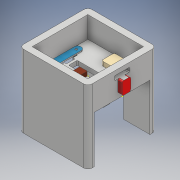
# Autodesk Inventor part: parts of all
Saved by Autodesk Inventor 2018 (Build 220112000, 112)
## iProperties
Created: 2019-01-10
Part Number: parts of all
Material: Generic
Document SubType Name: Modeling
Designer: USER
Density: 1 g/cm^3
Appearance: Default
Author: USER
Autodesk Inventor part; units mm, degrees
ref_plane "YZ Plane" through (0, 0, 0) normal (1, 0, 0) x (0, 1, 0)
ref_plane "XZ Plane" through (0, 0, 0) normal (0, 1, 0) x (-1, 0, 0)
ref_plane "XY Plane" through (0, 0, 0) normal (0, 0, 1) x (1, 0, 0)
sketch "Sketch1" plane through (0, 0, 0) normal (0, 0, 1) x (1, 0, 0)
  line L0 (-80, -80) -> (80, -80)
  line L1 (80, -80) -> (80, 80)
  line L2 (80, 80) -> (-80, 80)
  line L3 (-80, 80) -> (-80, -80)
  line L4 (-80, -80) -> (80, 80) construction
  line L5 (80, -80) -> (-80, 80) construction
  point P0 (0, 0)
  dimension "d0" = 160
  dimension "d1" = 160
  constraints: 12 end point, 2 midpoint, 2 parallel, 1 horizontal, 1 perpendicular
  measures "d0" distance of L2.end L1.end
  measures "d1" distance of L1.end L0.end
extrude "Extrusion1" add sketch "Sketch1" along normal blind 60
sketch "Sketch2" plane through (0, 0, 60) normal (0, 0, 1) x (1, 0, 0)
  line L0 (-65, 65) -> (65, 65)
  line L1 (65, 65) -> (65, -65)
  line L2 (65, -65) -> (-65, -65)
  line L3 (-65, -65) -> (-65, 65)
  point P0 (0, 0)
  point P1 (-80, 80)
  point P2 (-80, -80)
  point P3 (80, -80)
  constraints: 8 end point, 2 parallel, 1 horizontal, 1 perpendicular
extrude "Extrusion2" cut sketch "Sketch2" against normal blind 50
sketch "Sketch18" plane through (0, 0, 0) normal (0, 0, -1) x (-1, 0, 0)
  line L0 (80, 80) -> (80, -80)
  line L1 (80, 80) -> (80, -80) projected
  line L2 (45, 20) -> (65, 20)
  line L3 (65, 20) -> (65, -20)
  line L4 (65, -20) -> (45, -20)
  line L5 (45, -20) -> (45, 20)
  line L6 (45, 20) -> (65, -20) construction
  line L7 (65, 20) -> (45, -20) construction
  point P0 (0, 0)
  dimension "d40" = 20
  dimension "d41" = 40
  constraints: 14 end point, 2 parallel, 1 horizontal, 1 perpendicular
  measures "d40" distance of L3.end L4.end
  measures "d41" distance of L2.end L3.end
extrude "Extrusion5" cut sketch "Sketch18" against normal blind 20
sketch "Sketch26" plane through (-78, 80, 0) normal (0, 1, 0) x (1, 0, 0)
  line L0 (143, -12) -> (143, -18) projected
  line L1 (143, -15) -> (113, -15)
  line L2 (113, -15) -> (113, -25)
  line L3 (113, -25) -> (143, -25)
  line L4 (143, -25) -> (143, -15)
  point P0 (78, 0)
  dimension "d65" = 30
  dimension "d66" = 10
  constraints: 8 end point, 2 parallel, 1 horizontal, 1 midpoint, 1 perpendicular
  measures "d65" distance of L3.end L2.end
  measures "d66" distance of L2.end L1.end
extrude "Extrusion9" cut sketch "Sketch26" against normal blind 20
fillet "Fillet4" radius 2 4 edges at (65, 72.5, 25) (65, 72.5, 15) (35, 72.5, 25) (35, 72.5, 15)
sketch "Sketch36" plane through (0, 0, 10) normal (0, 0, 1) x (1, 0, 0)
  line L0 (0, -10) -> (35, -10)
  line L1 (35, -10) -> (35, 0)
  line L2 (-35, 10) -> (35, 10)
  line L3 (35, 10) -> (35, -10)
  line L4 (35, -10) -> (-35, -10)
  line L5 (-35, -10) -> (-35, 10)
  line L6 (-35, 10) -> (35, -10) construction
  line L7 (35, 10) -> (-35, -10) construction
  point P0 (0, 0)
  dimension "d75" = 10
  dimension "d76" = 35
  dimension "d77" = 10
  constraints: 16 end point, 2 midpoint, 2 parallel, 2 perpendicular, 1 horizontal
  measures "d75" distance of point (0, 0) L0.start
  measures "d76" distance of L0.start L0.end
  measures "d77" distance of L0.end L1.end
extrude "Extrusion11" cut sketch "Sketch36" against normal blind 20
sketch "Sketch37" plane through (0, 0, 10) normal (0, 0, 1) x (1, 0, 0)
  line L0 (-49.7695, 10) -> (-40.2305, 10)
  line L1 (-40.2305, 10) -> (-40.2305, -10)
  line L2 (-40.2305, -10) -> (-49.7695, -10)
  line L3 (-49.7695, -10) -> (-49.7695, 10)
  line L4 (-45, 20) -> (-45, -20) projected
  line L5 (-49.7695, 10) -> (-40.2305, -10) construction
  line L6 (-40.2305, 10) -> (-49.7695, -10) construction
  point P0 (0, 0)
  point P1 (-45, 0)
  point P2 (-45, 18)
  point P3 (-45, -18)
  constraints: 12 end point, 3 midpoint, 2 parallel, 1 horizontal, 1 perpendicular
extrude "Extrusion12" cut sketch "Sketch37" against normal blind 20
fillet "Fillet6" radius 2 4 edges at (35, 10, 5) (35, -10, 5) (-35, -10, 5) (-35, 10, 5)
fillet "Fillet7" radius 10 4 edges at (80, 80, 30) (-80, 80, 30) (-80, -80, 30) (80, -80, 30)
fillet "Fillet8" radius 2 2 edges at (-40.2305, 10, 5) (-40.2305, -10, 5)
sketch "Sketch46" plane through (0, 0, 10) normal (0, 0, 1) x (1, 0, 0)
  line L0 (-65, 20) -> (-45, 20) projected
  line L1 (-45, 20) -> (-45, 21)
  line L2 (-45, -20) -> (-45, -10) projected
  line L3 (-45, -20) -> (-45, -21)
  line L4 (-45, -21) -> (-65, -21)
  line L5 (-65, -21) -> (-65, -20)
  line L6 (-65, -20) -> (-45, -20)
  line L7 (-45, -20) -> (-45, -21)
  line L8 (-45, 21) -> (-65, 21)
  line L9 (-65, 21) -> (-65, 20)
  line L10 (-65, 20) -> (-45, 20)
  line L11 (-45, 20) -> (-45, 21)
  point P0 (0, 0)
  dimension "d87" = 1
  dimension "d88" = 1
  dimension "d89" = 20
  dimension "d90" = 1
  dimension "d91" = 20
  dimension "d92" = 1
  constraints: 20 end point, 4 parallel, 2 horizontal, 2 perpendicular, 2 vertical
  measures "d87" distance of L0.end L1.end
  measures "d88" distance of L2.start L3.end
  measures "d89" distance of L5.end L6.end
  measures "d90" distance of L4.end L5.end
  measures "d91" distance of L10.end L0.start
  measures "d92" distance of L0.start L8.end
extrude "Extrusion13" cut sketch "Sketch46" against normal blind 10
fillet "Fillet9" radius 2 4 edges at (-45, 21, 5) (-65, 21, 5) (-65, -21, 5) (-45, -21, 5)
sketch "Sketch51" plane through (80, -70, 0) normal (1, 0, 0) x (0, 0, -1)
  line L0 (-60, 5) -> (-60, 135) projected
  line L1 (-60, 70) -> (-45, 70)
  line L2 (-50, 52.5) -> (-40, 52.5)
  line L3 (-40, 52.5) -> (-40, 87.5)
  line L4 (-40, 87.5) -> (-50, 87.5)
  line L5 (-50, 87.5) -> (-50, 52.5)
  line L6 (-50, 52.5) -> (-40, 87.5) construction
  line L7 (-40, 52.5) -> (-50, 87.5) construction
  point P0 (0, 70)
  dimension "d103" = 15
  dimension "d104" = 10
  dimension "d105" = 35
  constraints: 14 end point, 3 midpoint, 2 horizontal, 2 parallel, 1 perpendicular
  measures "d103" distance of L1.start L1.end
  measures "d104" distance of L4.end L3.end
  measures "d105" distance of L3.end L2.end
extrude "Extrusion14" cut sketch "Sketch51" against normal blind 30
fillet "Fillet10" radius 2 4 edges at (72.5, -17.5, 40) (72.5, -17.5, 50) (72.5, 17.5, 40) (72.5, 17.5, 50)
sketch "Sketch67" plane through (80, -70, 60) normal (1, 0, 0) x (0, 0, -1)
  line L0 (50, 60) -> (20, 60)
  line L1 (20, 60) -> (20, 80)
  line L2 (20, 80) -> (50, 80)
  line L3 (50, 80) -> (50, 60)
  point P0 (60, 70)
  point P1 (60, 60)
  dimension "d130" = 10
  dimension "d131" = 30
  dimension "d132" = 20
  constraints: 8 end point, 2 parallel, 1 horizontal, 1 perpendicular
  measures "d130" distance of point (60, 60) L0.start
  measures "d131" distance of L1.end L2.end
  measures "d132" distance of L0.end L1.end
extrude "Extrusion17" add sketch "Sketch67" along normal blind 10
fillet "Fillet15" radius 4 4 edges at (85, -10, 10) (85, 10, 10) (85, 10, 40) (85, -10, 40)
sketch "Sketch68" plane through (80, -70, 60) normal (1, 0, 0) x (0, 0, -1)
  point P0 (60, 70)
sketch "Sketch69" plane through (0, 0, 10) normal (0, 0, 1) x (1, 0, 0)
  line L0 (58.5126, 28.0445) -> (3.5126, 28.0445)
  line L1 (3.5126, 28.0445) -> (3.5126, 58.0445)
  line L2 (3.5126, 58.0445) -> (58.5126, 58.0445)
  line L3 (58.5126, 58.0445) -> (58.5126, 28.0445)
  point P0 (0, 0)
  dimension "d136" = 55
  dimension "d137" = 30
  constraints: 8 end point, 2 parallel, 1 horizontal, 1 perpendicular
  measures "d136" distance of L1.end L2.end
  measures "d137" distance of L0.end L1.end
extrude "Extrusion18" add sketch "Sketch69" along normal blind 10
fillet "Fillet16" radius 4 4 edges at (3.5126, 28.0445, 15) (3.5126, 58.0445, 15) (58.5126, 58.0445, 15) (58.5126, 28.0445, 15)
sketch "Sketch70" plane through (80, -10, 14) normal (0, -1, 0) x (1, 0, 0)
  point P0 (-80, -14)
sketch "Sketch78" plane through (0, 0, 10) normal (0, 0, 1) x (1, 0, 0)
  line L0 (33, -10) -> (-33, -10) projected
  line L1 (8.7053, -27.8361) -> (-9.0694, -27.8361)
  line L2 (-9.0694, -27.8361) -> (-9.0694, -10)
  line L3 (-9.0694, -10) -> (8.7053, -10)
  line L4 (8.7053, -10) -> (8.7053, -27.8361)
  point P0 (0, 0)
  constraints: 8 end point, 2 parallel, 1 horizontal, 1 perpendicular, 1 point on line
extrude "Extrusion23" add sketch "Sketch78" along normal blind 10
sketch "Sketch79" plane through (0, 0, 10) normal (0, 0, 1) x (1, 0, 0)
  line L0 (-54.8796, -27.6723) -> (-54.8796, 31.1604) construction
  line L1 (-46.9698, -27.6723) -> (-46.9698, 31.1604)
  line L2 (-62.7894, 31.1604) -> (-62.7894, -27.6723)
  arc A0 (-62.7894, -27.6723) -> (-46.9698, -27.6723) centre (-54.8796, -27.6723) ccw
  arc A1 (-46.9698, 31.1604) -> (-62.7894, 31.1604) centre (-54.8796, 31.1604) ccw
  point P0 (0, 0)
  point P1 (-54.8796, 1.7441)
  constraints: 8 end point, 4 point on circle, 4 tangent, 2 centre point, 1 midpoint, 1 parallel, 1 vertical
extrude "Extrusion24" add sketch "Sketch79" along normal blind 3
sketch "Sketch83" plane through (0, 0, 0) normal (0, 0, -1) x (-1, 0, 0)
  circle A0 centre (54.5538, -27.479) radius 2.5
  point P0 (0, 0)
  dimension "d161" = 5
  constraints: 1 centre point
  measures "d161" diameter of A0
extrude "Extrusion26" cut sketch "Sketch83" against normal blind 30
sketch "Sketch86" plane through (0, 0, 0) normal (0, 0, -1) x (-1, 0, 0)
  point P0 (0, 0)
sketch "Sketch88" plane through (0, 0, 0) normal (0, 0, -1) x (-1, 0, 0)
  circle A0 centre (55, 28.399) radius 2.5
  point P0 (0, 0)
  dimension "d165" = 5
  constraints: 1 centre point
  measures "d165" diameter of A0
extrude "Extrusion27" cut sketch "Sketch88" against normal blind 30
sketch "Sketch91" plane through (0, 0, 0) normal (0, 0, -1) x (-1, 0, 0)
  line L0 (-80, 80) -> (80, 80)
  line L1 (80, 80) -> (80, 65)
  line L2 (80, 65) -> (-80, 65)
  line L3 (-80, 65) -> (-80, 80)
  point P0 (0, 0)
  dimension "d168" = 160
  dimension "d169" = 15
  constraints: 8 end point, 2 parallel, 1 horizontal, 1 perpendicular
  measures "d168" distance of L1.end L2.end
  measures "d169" distance of L0.end L1.end
extrude "Extrusion28" add sketch "Sketch91" along normal blind 110
sketch "Sketch92" plane through (0, 0, 0) normal (0, 0, -1) x (-1, 0, 0)
  line L0 (80, -80) -> (-80, -80)
  line L1 (-80, -80) -> (-80, -65)
  line L2 (-80, -65) -> (80, -65)
  line L3 (80, -65) -> (80, -80)
  point P0 (0, 0)
  dimension "d172" = 160
  dimension "d173" = 15
  constraints: 8 end point, 2 parallel, 1 horizontal, 1 perpendicular
  measures "d172" distance of L1.end L2.end
  measures "d173" distance of L0.end L1.end
extrude "Extrusion29" add sketch "Sketch92" along normal blind 110
fillet "Fillet17" radius 10 2 edges at (80, 80, -55) (-80, 80, -55)
sketch "Sketch97" plane through (-70, 80, 60) normal (0, 1, 0) x (1, 0, 0)
  line L0 (0, 170) -> (140, 170) projected
  line L1 (88.0594, 170) -> (40.976, 170)
  line L2 (40.976, 170) -> (40.976, 99.9886)
  line L3 (40.976, 99.9886) -> (88.0594, 99.9886)
  line L4 (88.0594, 99.9886) -> (88.0594, 170)
  point P0 (70, 60)
  constraints: 8 end point, 2 parallel, 1 horizontal, 1 perpendicular, 1 point on line
extrude "Extrusion31" cut sketch "Sketch97" against normal blind 110
fillet "Fillet18" radius 10 2 edges at (80, -80, -55) (-80, -80, -55)
body "Solid1"
